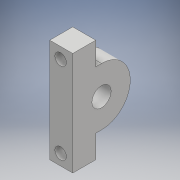
# Autodesk Inventor part: attachment
Saved by Autodesk Inventor 2017 (Build 210142000, 142)
## iProperties
Created: 2017-04-28
Part Number: attachment
Material: Generic
Document SubType Name: Modeling
Designer: s4321966
Density: 1 g/cm^3
Appearance: Default
Author: s4321966
Autodesk Inventor part; units mm, degrees
ref_plane "YZ Plane" through (0, 0, 0) normal (1, 0, 0) x (0, 1, 0)
ref_plane "XZ Plane" through (0, 0, 0) normal (0, 1, 0) x (-1, 0, 0)
ref_plane "XY Plane" through (0, 0, 0) normal (0, 0, 1) x (1, 0, 0)
sketch "Sketch1" plane through (0, 0, 0) normal (1, 0, 0) x (0, 1, 0)
  circle A0 centre (0, 0) radius 1.25
  circle A1 centre (0, 0) radius 3.75
  line L0 (0, -3.75) -> (-3.5355, -3.75)
  line L1 (-3.5355, -3.75) -> (-3.5355, -1.25)
  line L2 (-3.5355, -1.25) -> (0, -1.25)
  line L3 (0, -1.25) -> (0, -3.75)
  line L4 (0, 3.75) -> (-2.9201, 3.75)
  line L5 (-2.9201, 3.75) -> (-2.9201, 1.25)
  line L6 (-2.9201, 1.25) -> (0, 1.25)
  line L7 (0, 1.25) -> (0, 3.75)
  line L8 (-3.75, 0) -> (-1.25, 0)
  line L9 (-1.25, 0) -> (-1.25, -3.75)
  line L10 (-1.25, -3.75) -> (-3.75, -3.75)
  line L11 (-3.75, -3.75) -> (-3.75, 0)
  line L12 (-3.75, 0) -> (-1.25, 0)
  line L13 (-1.25, 0) -> (-1.25, 3.75)
  line L14 (-1.25, 3.75) -> (-3.75, 3.75)
  line L15 (-3.75, 3.75) -> (-3.75, 0)
  line L16 (-3.75, 3.75) -> (-0.75, 3.75)
  line L17 (-0.75, 3.75) -> (-0.75, 6.75)
  line L18 (-0.75, 6.75) -> (-3.75, 6.75)
  line L19 (-3.75, 6.75) -> (-3.75, 3.75)
  line L20 (0, -3.75) -> (-2.9201, -3.75)
  line L21 (-0.75, -3.75) -> (-0.75, -6.75)
  line L22 (-0.75, -6.75) -> (-3.75, -6.75)
  line L23 (-3.75, -6.75) -> (-3.75, -3.75)
  line L24 (-0.75, -6.75) -> (-3.75, -6.75)
  line L25 (-3.75, -6.75) -> (-3.75, -3.75)
  line L26 (-3.75, -3.75) -> (-0.75, -3.75)
  line L27 (-0.75, -3.75) -> (-0.75, -6.75)
  dimension "d0" = 2.5
  dimension "d1" = 7.5
  dimension "d2" = 3
  dimension "d3" = 3
  constraints: 56 end point, 12 parallel, 6 horizontal, 6 perpendicular, 4 point on circle, 4 point on line, 4 symmetric about line, 2 centre point, 2 coincident
  measures "d0" diameter of A0
  measures "d1" diameter of A1
  measures "d2" distance of L18.end L17.end
  measures "d3" distance of L17.end L16.end
extrude "Extrusion1" add sketch "Sketch1" along normal blind 3
sketch "Sketch2" plane through (3, 0, 0) normal (1, 0, 0) x (0, 0, -1)
  circle A0 centre (0, 0) radius 1.25
  dimension "d6" = 2.5
  constraints: 1 centre point, 1 coincident
  measures "d6" diameter of A0
extrude "Extrusion2" cut sketch "Sketch2" against normal blind 10
sketch "Sketch3" plane through (0, -0.75, 6.75) normal (0, 1, 0) x (1, 0, 0)
  line L0 (0, 0) -> (3, 3.0493)
  line L1 (3, 0) -> (3, 13.5) projected
  line L2 (0, 6.75) -> (4.6316, 6.75)
  circle A0 centre (1.4195, 1.4429) radius 0.75
  line L3 (0, 13.5) -> (3, 10.4507)
  circle A1 centre (1.4195, 12.0571) radius 0.75
  dimension "d9" = 1.5
  constraints: 6 end point, 3 point on line, 3 symmetric about line, 2 centre point, 1 horizontal, 1 other
  measures "d9" diameter of A0
extrude "Extrusion3" cut sketch "Sketch3" against normal blind 10
body "Solid1"
